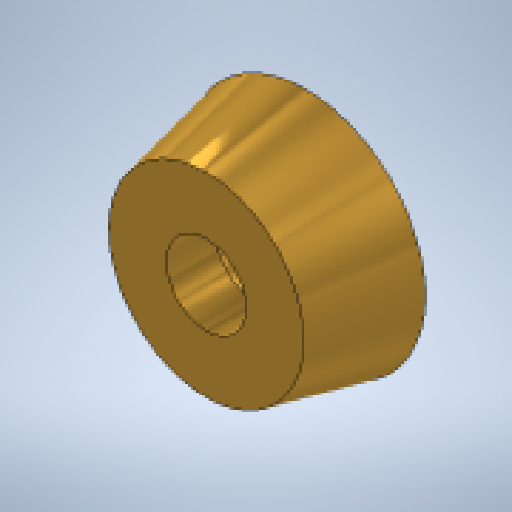
# Autodesk Inventor part: Flywheel
Saved by Autodesk Inventor 2023.2 (Build 272271000, 271)
## iProperties
Created: 2024-03-17
Part Number: Flywheel
Material: Brass, Soft Yellow
Document SubType Name: Modeling
Designer: Nathan Cai
Mass: 25.2582 g
Surface Area: 38.7806 cm^2
Volume: 2.98207 cm^3
Density: 8.47 g/cm^3
Appearance: Brass - Satin
Author: Nathan Cai
Autodesk Inventor part; units mm, degrees
ref_plane "YZ Plane" through (0, 0, 0) normal (1, 0, 0) x (0, 1, 0)
ref_plane "XZ Plane" through (0, 0, 0) normal (0, 1, 0) x (-1, 0, 0)
ref_plane "XY Plane" through (0, 0, 0) normal (0, 0, 1) x (1, 0, 0)
sketch "Sketch1" plane through (0, 0, 0) normal (1, 0, 0) x (0, 1, 0)
  line L0 (0, 0) -> (13.95, 0) construction
  line L1 (13.95, 0) -> (13.95, 8)
  line L2 (13.95, 8) -> (0, 8)
  line L3 (0, 8) -> (0, 0) construction
  line L4 (0, 8) -> (6.35, 8)
  line L5 (6.35, 8) -> (6.35, 13.55)
  line L6 (6.35, 13.55) -> (0, 13.55) construction
  line L7 (0, 13.55) -> (0, 8) construction
  line L8 (0, 0) -> (15.875, 0)
  line L9 (15.875, 0) -> (15.875, 13.55)
  line L10 (15.875, 13.55) -> (0, 13.55)
  line L11 (0, 13.55) -> (0, 0)
  line L12 (13.7634, 13.55) -> (15.875, 4.025)
  line L13 (6.35, 8) -> (5.35, 8)
  line L14 (5.35, 8) -> (5.35, 9.5813)
  line L15 (5.35, 9.5813) -> (6.35, 9.5813)
  line L16 (6.35, 9.5813) -> (6.35, 8)
  line L17 (12.7, 13.55) -> (7.9375, 13.55)
  line L18 (7.9375, 13.55) -> (7.9375, 9.5875)
  line L19 (7.9375, 9.5875) -> (12.7, 9.5875)
  line L20 (12.7, 9.5875) -> (12.7, 13.55)
  point P0 (13.95, 0)
  point P1 (0, 8)
  point P2 (6.35, 9.5813)
  dimension "d0" = 13.95
  dimension "d1" = 8
  dimension "d2" = 6.35
  dimension "d3" = 13.55
  dimension "d4" = 15.875
  dimension "d7" = 12.5
  dimension "d8" = 9.525
  dimension "d9" = 1
  dimension "d10" = 3.9688
  dimension "d17" = 1.5875
  dimension "d18" = 1.5875
  dimension "d19" = 3.175
  constraints: 42 end point, 10 parallel, 5 horizontal, 5 perpendicular, 4 point on line
  measures "d0" distance of L2.end L1.end
  measures "d1" distance of L1.end L0.end
  measures "d2" distance of L6.end L5.end
  measures "d3" distance between parallel lines of L0 L6
  measures "d4" distance between parallel lines of L3 L9
  measures "d7" angle of L9 L12
  measures "d8" distance from line of L10 L12.end
  measures "d9" distance of L14.end L15.end
  measures "d10" distance between parallel lines of L10 L15
  measures "d17" distance between parallel lines of L5 L18
  measures "d18" distance between parallel lines of L2 L19
  measures "d19" distance between parallel lines of L9 L20
revolve "Revolution1" add sketch "Sketch1" angle 360 about axis through (0, 0, 13.55) along (0, 0, -1) contours L1 L2 L5 L10 L18 L19 L20 L12 L9 L8 | L2 L14 L15 L5
chamfer "Chamfer2" distance 0.5 angle 45 4 edges at (0, -6.35, 13.55) (0, -15.875, 0) (0, -5.35, 8) (0, -7.9375, 13.55)
body "Solid1"
